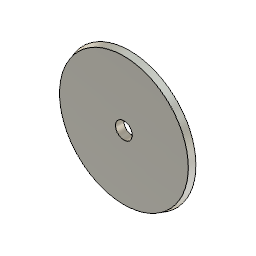
Ensamble v3 (Autodesk Fusion 360 archive; units mm, degrees)
design "Anillo de engrane 2"
Autodesk Fusion 360 part; units mm, degrees
sketch "Boceto1" plane through (0, 0, 0) normal (0, 0, 1) x (1, 0, 0)
  line L0 (0, 0) -> (17.25, 0)
  line L1 (17.25, 0) -> (17.7374, 1.5868)
  line L2 (17.7374, 1.5868) -> (15.6725, 2.221)
  line L3 (15.6725, 2.221) -> (0, 2.221)
  line L4 (0, 2.221) -> (0, 0)
  line L5 (0, 1.5868) -> (17.7374, 1.5868) construction
  dimension "d1" = 17.25
  dimension "d3" = 1.66
  dimension "d4" = 2.16
  dimension "d16" = 90
  dimension "d22" = 2.221
  constraint coincident L0.start L4.end
  constraint horizontal L0
  constraint parallel L0 L3
  constraint perpendicular L0 L4
  constraint coincident L4 L5.start
  constraint perpendicular L4 L5
  measures "d1" distance of L0.start L0.end
  measures "d3" distance of L0.end L1.end
  measures "d4" distance of L1.end L2.end
  measures "d16" angle of L1 L2
  measures "d22" distance of L0 L3
revolve "Revolución2" add sketch "Boceto1" angle 360 about axis through (0, 2.221, 0) along (0, -1, 0)
sketch "Boceto4" plane through (0, 0, 0) normal (0, -1, 0) x (1, 0, 0)
  circle A0 centre (0, 0) radius 17.25
  circle A1 centre (0, 0) radius 2.25
  dimension "d19" = 4.5
  constraint coincident A0.centre A1.centre
  measures "d19" diameter of A1
extrude "Extruir3" cut sketch "Boceto4" along normal mid plane 26 contours A1

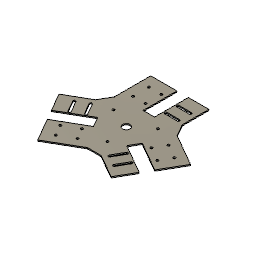
design "Robot Delta base"
Autodesk Fusion 360 part; units mm, degrees
sketch "Boceto1" plane through (0, 0, 0) normal (0, 0, 1) x (1, 0, 0)
  circle A0 centre (0, 0) radius 100
  line L0 (0, 200.0885) -> (-173.2817, -100.0442)
  line L1 (-173.2817, -100.0442) -> (173.2817, -100.0442)
  line L2 (173.2817, -100.0442) -> (0, 200.0885)
  line L3 (0, -100.0442) -> (0, 200.0885) construction
  line L4 (-173.2817, -100.0442) -> (86.6408, 50.0221) construction
  line L5 (173.2817, -100.0442) -> (-86.6408, 50.0221) construction
  line L6 (51.9615, -30) -> (59.4615, -17.0096)
  line L7 (59.4615, -17.0096) -> (128.7436, -57.0096)
  line L8 (44.4615, -42.9904) -> (113.7436, -82.9904)
  line L9 (51.9615, -30) -> (44.4615, -42.9904)
  line L10 (-15, 60) -> (-15, 140)
  line L11 (0.5917, 60) -> (15, 60)
  line L12 (15, 60) -> (15, 140)
  line L13 (-123.1844, 140) -> (49.0279, 140)
  line L14 (-15, 60) -> (0.5917, 60)
  line L15 (157.2934, 41.8591) -> (75.3655, -100.0442)
  line L16 (-44.4615, -42.9904) -> (-113.7436, -82.9904)
  line L17 (-59.4615, -17.0096) -> (-128.7436, -57.0096)
  line L18 (-30.9577, -176.4773) -> (-124.184, -15.0046)
  line L19 (-44.4615, -42.9904) -> (-59.4615, -17.0096)
  circle A1 centre (0, 0) radius 10
  line L20 (-115.5498, 0.1381) -> (-24.8334, -156.9872) construction
  line L21 (212.8999, -69.8468) -> (210.5798, -60.2903) construction
  line L22 (57.7095, -100.0442) -> (164.8904, 85.5986) construction
  line L23 (57.7861, 100) -> (-125, 100) construction
  line L24 (-85, 150) -> (-15, 150)
  line L25 (-15, 150) -> (-15, 50)
  line L26 (-15, 50) -> (-85, 50)
  line L27 (-85, 50) -> (-85, 150)
  circle A2 centre (45, 84) radius 3
  circle A3 centre (25, 84) radius 3
  circle A4 centre (25, 116) radius 3
  circle A5 centre (45, 116) radius 3
  line L28 (28.8663, 150.0905) -> (70, 150.0905)
  line L29 (70, 150.0905) -> (70, 78.8449)
  line L30 (21, 113) -> (55, 113)
  line L31 (21, 119) -> (55, 119)
  arc A6 (55, 113) -> (55, 119) centre (55, 116) ccw
  arc A7 (21, 119) -> (21, 113) centre (21, 116) ccw
  line L32 (21, 81) -> (55, 81)
  circle A8 centre (25, 84) radius 3
  circle A9 centre (45, 84) radius 3
  line L33 (21, 87) -> (55, 87)
  arc A10 (21, 87) -> (21, 81) centre (21, 84) ccw
  arc A11 (55, 81) -> (55, 87) centre (55, 84) ccw
  line L34 (-0.8013, -98.6122) -> (-87.4038, -148.6122)
  line L35 (-35.8013, -37.9904) -> (-0.8013, -98.6122)
  line L36 (-44.4615, -42.9904) -> (-113.7436, -82.9904)
  line L37 (-122.4038, -87.9904) -> (-35.8013, -37.9904)
  line L38 (-87.4038, -148.6122) -> (-122.4038, -87.9904)
  line L39 (-59.6514, -176.6808) -> (-145.7575, -27.5406)
  line L40 (-59.4615, -17.0096) -> (-128.7436, -57.0096)
  line L41 (-52.2574, -29.4875) -> (-59.4615, -17.0096)
  line L42 (-44.4615, -42.9904) -> (-52.2574, -29.4875)
  line L43 (-80.6481, -22.3135) -> (-97.6481, 7.1314)
  circle A12 centre (-112.9589, -36.3494) radius 3
  circle A13 centre (-122.9589, -19.0289) radius 3
  circle A14 centre (-85.2461, -20.3494) radius 3
  circle A15 centre (-95.2461, -3.0289) radius 3
  line L44 (-85.8442, -25.3135) -> (-102.8442, 4.1314)
  arc A16 (-85.8442, -25.3135) -> (-80.6481, -22.3135) centre (-83.2461, -23.8135) ccw
  arc A17 (-97.6481, 7.1314) -> (-102.8442, 4.1314) centre (-100.2461, 5.6314) ccw
  arc A18 (-113.557, -41.3135) -> (-108.3609, -38.3135) centre (-110.9589, -39.8135) ccw
  line L45 (-108.3609, -38.3135) -> (-125.3609, -8.8686)
  line L46 (-113.557, -41.3135) -> (-130.557, -11.8686)
  arc A19 (-125.3609, -8.8686) -> (-130.557, -11.8686) centre (-127.9589, -10.3686) ccw
  line L47 (-144.4154, -50.0463) -> (-164.9822, -14.4235)
  line L48 (-164.9822, -14.4235) -> (-103.2817, 21.1993)
  line L49 (85.8013, 48.6122) -> (172.4038, -1.3878)
  line L50 (50.8013, -12.0096) -> (85.8013, 48.6122)
  line L51 (59.4615, -17.0096) -> (128.7436, -57.0096)
  line L52 (137.4038, -62.0096) -> (50.8013, -12.0096)
  line L53 (172.4038, -1.3878) -> (137.4038, -62.0096)
  line L54 (182.8357, 36.6808) -> (96.7296, -112.4594)
  line L55 (44.4615, -42.9904) -> (113.7436, -82.9904)
  line L56 (51.6657, -30.5125) -> (44.4615, -42.9904)
  line L57 (59.4615, -17.0096) -> (51.6657, -30.5125)
  line L58 (59.6481, -58.6865) -> (42.6481, -88.1314)
  circle A20 centre (87.9589, -79.6506) radius 3
  circle A21 centre (77.9589, -96.9711) radius 3
  circle A22 centre (60.2461, -63.6506) radius 3
  circle A23 centre (50.2461, -80.9711) radius 3
  line L59 (64.8442, -61.6865) -> (47.8442, -91.1314)
  arc A24 (64.8442, -61.6865) -> (59.6481, -58.6865) centre (62.2461, -60.1865) ccw
  arc A25 (42.6481, -88.1314) -> (47.8442, -91.1314) centre (45.2461, -89.6314) ccw
  arc A26 (92.557, -77.6865) -> (87.3609, -74.6865) centre (89.9589, -76.1865) ccw
  line L60 (87.3609, -74.6865) -> (70.3609, -104.1314)
  line L61 (92.557, -77.6865) -> (75.557, -107.1314)
  arc A27 (70.3609, -104.1314) -> (75.557, -107.1314) centre (72.9589, -105.6314) ccw
  line L62 (115.549, -100.0442) -> (94.9822, -135.667)
  line L63 (94.9822, -135.667) -> (33.2817, -100.0442)
  line L64 (-15, 150) -> (28.8663, 150.0905)
  line L65 (15, 150.0619) -> (15, 140)
  line L66 (-144.4154, -50.0463) -> (-122.4038, -87.9904)
  line L67 (115.549, -100.0442) -> (137.4038, -62.0096)
  line L68 (122.3417, -88.2227) -> (113.7436, -82.9904)
  line L69 (-137.4729, -62.0138) -> (-128.7436, -57.0096)
  circle A28 centre (118.8973, -36.3138) radius 3
  circle A29 centre (135.4123, -7.709) radius 3
  circle A30 centre (98.8228, 13.416) radius 3
  circle A31 centre (82.3078, -15.1888) radius 3
  circle A32 centre (-61.03, 121.125) radius 3
  circle A33 centre (-28, 121.125) radius 3
  circle A34 centre (-28, 78.875) radius 3
  circle A35 centre (-61.03, 78.875) radius 3
  circle A36 centre (-74.3823, -113.416) radius 3
  circle A37 centre (-90.8973, -84.8112) radius 3
  circle A38 centre (-54.3078, -63.6862) radius 3
  circle A39 centre (-37.7928, -92.291) radius 3
  line L70 (-3.1207, -99.9513) -> (33.2817, -100.0442)
  line L71 (-103.2817, 21.1993) -> (-85, 52.8641)
  line L72 (0, 0) -> (15.0803, -100.0442) construction
  circle A40 centre (8.9431, -59.3298) radius 3
  circle A41 centre (0, 0) radius 60 construction
  circle A42 centre (46.9095, 37.4099) radius 3
  circle A43 centre (-55.8526, 21.9199) radius 3
  point P0 (-86.6025, -50)
  point P1 (-85.2461, -20.3494)
  point P2 (60.2461, -63.6506)
  dimension "d1" = 200
  dimension "d5" = 80
  dimension "d6" = 60
  dimension "d7" = 30
  dimension "d8" = 80
  dimension "d9" = 30
  dimension "d10" = 15
  dimension "d13" = 60
  dimension "d16" = 80
  dimension "d17" = 30
  dimension "d18" = 15
  dimension "d19" = 60
  dimension "d22" = 80
  dimension "d24" = 80
  dimension "d25" = 20
  dimension "d27" = 70
  dimension "d28" = 100
  dimension "d29" = 50
  dimension "d47" = 6
  dimension "d48" = 6
  dimension "d49" = 6
  dimension "d50" = 6
  dimension "d51" = 20
  dimension "d52" = 20
  dimension "d53" = 32
  dimension "d55" = 10
  dimension "d56" = 10
  dimension "d57" = 16
  dimension "d58" = 16
  dimension "d59" = 32
  dimension "d60" = 10
  dimension "d61" = 4
  dimension "d62" = 4
  dimension "d63" = 10
  dimension "d68" = 6
  dimension "d69" = 13
  dimension "d70" = 21.125
  dimension "d71" = 6
  dimension "d72" = 33.03
  dimension "d73" = 21.125
  dimension "d74" = 21.125
  dimension "d76" = 360
  dimension "d94" = 36.4024
  dimension "d95" = 18.201
  dimension "d96" = 6
  dimension "d98" = 60
  dimension "d99" = 120
  dimension "d101" = 360
  constraint coincident A0.centre A1.centre
  constraint midpoint L1 L3.start
  constraint perpendicular L1 L3
  constraint midpoint L2 L4.end
  constraint perpendicular L2 L4
  constraint midpoint L0 L5.end
  constraint perpendicular L0 L5
  constraint coincident L5 L6.start
  constraint perpendicular L5 L6
  constraint perpendicular L6 L7
  constraint symmetric L5 L6.start L9.start
  constraint symmetric L5 L6.end L8.start
  constraint symmetric L5 L7.end L8.end
  constraint perpendicular L12 L13
  constraint perpendicular L3 L14
  constraint perpendicular L17 L18
  constraint perpendicular L17 L19
  constraint horizontal L13
  constraint coincident L0 L18.end
  constraint coincident L1 L15.end
  constraint coincident A0 P0
  constraint coincident L4 P0
  constraint perpendicular L4 L20
  constraint tangent A0 L20
  constraint perpendicular L5 L22
  constraint tangent A0 L22
  constraint coincident L1 L22.start
  constraint equal L10 L12
  constraint coincident L2 L23.start
  constraint perpendicular L12 L23
  constraint horizontal L24
  constraint vertical L25
  constraint horizontal L26
  constraint vertical L27
  constraint coincident L2 L28.start
  constraint parallel L13 L28
  constraint coincident L2 L29.end
  constraint perpendicular L28 L29
  constraint perpendicular L3 L30
  constraint tangent A4 L31
  constraint tangent L30 A6
  constraint tangent L31 A6
  constraint tangent L30 A7
  constraint symmetric L23 A4 A8
  constraint symmetric L23 A5 A9
  constraint symmetric L23 L30.start L33.start
  constraint symmetric L23 L30.end L33.end
  constraint symmetric L23 L31.start L32.start
  constraint symmetric L23 L31.end L32.end
  constraint symmetric L23 A6 A11
  constraint symmetric L23 A7 A10
  constraint coincident L64 L65.start
  constraint perpendicular L13 L65
  constraint coincident L67 L68.start
  constraint coincident L66 L69.start
  constraint symmetric L22 A28 A31
  constraint symmetric L22 A29 A30
  constraint coincident A0 L70.start
  constraint coincident L34 L70.start
  constraint coincident L0 L71.end
  constraint coincident L27 L71.end
  constraint parallel L0 L71
  constraint coincident L1 L72.end
  constraint coincident L72 A40.centre
  constraint concentric A1 A41
  measures "d1" diameter of A0
  measures "d5" distance of L6.end L7.end
  measures "d6" distance of A0.centre L6.start
  measures "d7" distance of L7 L8
  measures "d8" distance of L10.start L10.end
  measures "d9" distance of L10 L12
  measures "d10" distance of L3 L12
  measures "d13" distance of A0.centre L14
  measures "d16" distance of L16.start L16.end
  measures "d17" distance of L16 L17
  measures "d18" distance of L4 L17
  measures "d19" distance of A0.centre L19
  measures "d22" distance of L17.start L17.end
  measures "d24" distance of L11 L13
  measures "d25" diameter of A1
  measures "d27" distance of L25 L27
  measures "d28" distance of L24.start L26.end
  measures "d29" distance of L23 L24
  measures "d47" diameter of A2
  measures "d48" diameter of A3
  measures "d49" diameter of A4
  measures "d50" diameter of A5
  measures "d51" distance of A2.centre A3.centre
  measures "d52" horizontal distance of A4.centre A5.centre
  measures "d53" vertical distance of A2.centre A5.centre
  measures "d55" distance of L12 A3.centre
  measures "d56" distance of L12 A4.centre
  measures "d57" distance of L23 A5.centre
  measures "d58" distance of L23 A4.centre
  measures "d59" distance of A3.centre A4.centre
  measures "d60" horizontal distance of A5.centre L30.end
  measures "d61" horizontal distance of A4.centre L30.start
  measures "d62" horizontal distance of A4.centre L31.start
  measures "d63" horizontal distance of A5.centre L31.end
  measures "d68" diameter of A28
  measures "d69" distance of L7 A28.centre
  measures "d70" distance of L22 A28.centre
  measures "d71" diameter of A29
  measures "d72" distance of A28.centre A29.centre
  measures "d73" distance of L22 A29.centre
  measures "d74" distance of L22 A30.centre
  measures "d94" horizontal distance of L63.end L70.start
  measures "d95" horizontal distance of L70.start L72.end
  measures "d96" diameter of A40
  measures "d98" distance of A0.centre A40.centre
  measures "d99" diameter of A41
extrude "Extruir3" add sketch "Boceto1" along normal blind 3 contours A0 L7 L49 L50 L51 L52 A30 | A0 L2 L7 L15 L49 L51 L52 A30 | A0 L1 L8 L15 L55 L59 A25 A26 L60 L70 | A0 L6 L8 L9 L11 L12 L14 L17 L19 L25 L26 L27 L32 L33 A10 A11 L34 L35 L37 L40 L41 L42 L43 L44 A16 A17 L49 L50 L52 L55 L56 L57 L58 L59 A24 A25 L70 | L2 L7 L15 L51 L52 L54 | A0 L2 L12 L13 L30 L31 A7 L33 A11 L49 | L1 L8 L15 L54 L55 A26 L61 | L2 L52 L53 L54 | L2 L15 L49 L54 | L2 L15 L49 | L1 L54 L67 L68 | L2 L49 L53 L54 | L2 L28 L29 L30 L31 A6 | L1 L60 L61 A27 L62 L63 | A0 L1 L16 L18 L34 L36 L37 A39 | A0 L16 L34 L35 L36 L37 A39 | A0 L10 L25 L26 L27 A35 | A0 L0 L10 L13 L25 L27 A35 | L2 L13 L64 L65 | L1 L18 L34 | L0 L13 L24 L25 | L1 L18 L34 L39 | L1 L16 L18 L36 L37 L39 | L0 L13 L24 L27 | L0 L13 L27 | L1 L34 L38 L39 | L1 L37 L38 L39 | A0 L0 L17 L18 L27 L40 L44 A17 A18 L45 L71 | L0 L17 L18 L39 L40 A18 L46 | L0 L45 L46 A19 L47 L48 | L0 L39 L66 L69

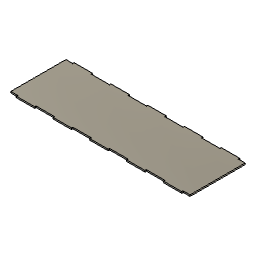
design "Parte Superior"
Autodesk Fusion 360 part; units mm, degrees
sketch "Boceto1" plane through (0, 0, 0) normal (0, 0, 1) x (1, 0, 0)
  line L0 (-195, 0) -> (-195, -60)
  line L1 (-100, -60) -> (-100, -63)
  line L2 (-100, -63) -> (-60, -63)
  line L3 (-60, -63) -> (-60, -60)
  line L4 (-60, -60) -> (-20, -60)
  line L5 (-20, -60) -> (-20, -63)
  line L6 (-20, -63) -> (0, -63)
  line L7 (0, 0) -> (-195, 0) construction
  line L8 (-100, 60) -> (-100, 63)
  line L9 (-100, 63) -> (-60, 63)
  line L10 (-20, 60) -> (-20, 63)
  line L11 (-60, 60) -> (-20, 60)
  line L12 (-60, 63) -> (-60, 60)
  line L13 (-20, 63) -> (0, 63)
  line L14 (-195, 0) -> (-195, 60)
  line L15 (0, -63) -> (0, 63) construction
  line L16 (0, -63) -> (0, 63) construction
  line L17 (-100, -60) -> (-140, -60)
  line L18 (-140, -60) -> (-140, -63)
  line L19 (-140, -63) -> (-180, -63)
  line L20 (-180, -63) -> (-180, -60)
  line L21 (-180, -60) -> (-195, -60)
  line L22 (-100, 60) -> (-140, 60)
  line L23 (-140, 60) -> (-140, 63)
  line L24 (-140, 63) -> (-180, 63)
  line L25 (-180, 63) -> (-180, 60)
  line L26 (-180, 60) -> (-195, 60)
  line L27 (60, -60) -> (20, -60)
  line L28 (100, 63) -> (60, 63)
  line L29 (60, 60) -> (20, 60)
  line L30 (0, 0) -> (195, 0) construction
  line L31 (20, 60) -> (20, 63)
  line L32 (20, 63) -> (0, 63)
  line L33 (140, -63) -> (180, -63)
  line L34 (180, -63) -> (180, -60)
  line L35 (180, -60) -> (195, -60)
  line L36 (195, 0) -> (195, -60)
  line L37 (195, 0) -> (195, 60)
  line L38 (180, 60) -> (195, 60)
  line L39 (180, 63) -> (180, 60)
  line L40 (140, 63) -> (180, 63)
  line L41 (100, -60) -> (140, -60)
  line L42 (100, -63) -> (60, -63)
  line L43 (20, -63) -> (0, -63)
  line L44 (100, 60) -> (140, 60)
  line L45 (140, 60) -> (140, 63)
  line L46 (100, -60) -> (100, -63)
  line L47 (140, -60) -> (140, -63)
  line L48 (20, -63) -> (20, -60)
  line L49 (60, -63) -> (60, -60)
  line L50 (100, 63) -> (100, 60)
  line L51 (60, 63) -> (60, 60)
  point P0 (0, 63)
  dimension "d2" = 195
  dimension "d4" = 20
  dimension "d6" = 40
  dimension "d7" = 3
  dimension "d8" = 3
  dimension "d9" = 3
  dimension "d10" = 60
  dimension "d13" = 40
  dimension "d14" = 40
  dimension "d15" = 3
  dimension "d16" = 40
  dimension "d17" = 3
  dimension "d18" = 40
  dimension "d19" = 3
  dimension "d20" = 40
  dimension "d21" = 3
  constraint vertical L0
  constraint perpendicular L1 L2
  constraint perpendicular L2 L3
  constraint perpendicular L3 L4
  constraint perpendicular L4 L5
  constraint perpendicular L5 L6
  constraint coincident L7.start L30.start
  constraint perpendicular L0 L7
  constraint symmetric L0.start L7 L14.start
  constraint symmetric L0.end L7 L14.end
  constraint symmetric L1.start L7 L8.start
  constraint symmetric L1.end L7 L8.end
  constraint symmetric L2.end L7 L9.end
  constraint symmetric L3.end L7 L11.start
  constraint symmetric L4.end L7 L10.start
  constraint symmetric L5.end L7 L10.end
  constraint symmetric P0 L15 L13.end
  constraint perpendicular L1 L17
  constraint perpendicular L17 L18
  constraint perpendicular L18 L19
  constraint perpendicular L19 L20
  constraint perpendicular L0 L21
  constraint perpendicular L8 L22
  constraint perpendicular L22 L23
  constraint perpendicular L23 L24
  constraint perpendicular L24 L25
  constraint symmetric L0.start L15 L30.end
  constraint symmetric L0.end L15 L35.end
  constraint symmetric L1.start L15 L41.start
  constraint symmetric L1.end L15 L42.start
  constraint symmetric L2.end L15 L42.end
  constraint symmetric L3.end L15 L27.start
  constraint symmetric L4.end L15 L27.end
  constraint symmetric L5.end L15 L43.start
  constraint symmetric L6.end L15 L16.start
  constraint symmetric L7.start L15 L30.start
  constraint symmetric L8.start L15 L44.start
  constraint symmetric L11.start L15 L29.start
  constraint symmetric L9.end L15 L28.end
  constraint symmetric L8.end L15 L28.start
  constraint symmetric L10.start L15 L29.end
  constraint symmetric L14.end L15 L37.end
  constraint symmetric L10.end L15 L31.end
  constraint symmetric L15 P0 L13.end
  constraint symmetric L15 L17.end L41.end
  constraint symmetric L15 L18.end L33.start
  constraint symmetric L15 L19.end L33.end
  constraint symmetric L15 L20.end L34.end
  constraint symmetric L15 L22.end L44.end
  constraint symmetric L15 L23.end L40.start
  constraint symmetric L15 L24.end L39.start
  constraint symmetric L15 L25.end L38.start
  measures "d2" distance of L0.start L7.start
  measures "d4" distance of L5.end L6.end
  measures "d6" distance of L1.end L2.end
  measures "d7" distance of L1.start L1.end
  measures "d8" distance of L2.end L3.end
  measures "d9" distance of L4.end L5.end
  measures "d10" distance of L0.start L0.end
  measures "d13" distance of L3.end L4.end
  measures "d14" distance of L1.start L17.end
  measures "d15" distance of L17.end L18.end
  measures "d16" distance of L18.end L19.end
  measures "d17" distance of L19.end L20.end
  measures "d18" distance of L8.start L22.end
  measures "d19" distance of L22.end L23.end
  measures "d20" distance of L23.end L24.end
  measures "d21" distance of L24.end L25.end
extrude "Extruir2" add sketch "Boceto1" along normal blind 3

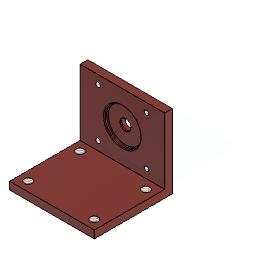
design "SoporteNEMA17 v10"
Autodesk Fusion 360 part; units mm, degrees
sketch "Sketch1" plane through (0, 0, 0) normal (0, 0, 1) x (1, 0, 0)
  line L0 (21.125, 21.125) -> (-21.125, 21.125)
  line L1 (-21.125, 21.125) -> (-21.125, -21.125)
  line L2 (-21.125, -21.125) -> (21.125, -21.125)
  line L3 (21.125, -21.125) -> (21.125, 21.125)
  line L4 (21.125, 21.125) -> (-21.125, -21.125) construction
  line L5 (-21.125, 21.125) -> (21.125, -21.125) construction
  dimension "d1" = 42.25
  dimension "d2" = 42.25
  constraint horizontal L0
  constraint perpendicular L0 L1
  constraint parallel L0 L2
  constraint parallel L1 L3
  constraint coincident L4 origin
  constraint coincident L5 origin
  measures "d1" distance of L1.end L2.end
  measures "d2" distance of L0.end L1.end
extrude "Extrude1" add sketch "Sketch1" along normal blind 5
sketch "Sketch2" plane through (0, 0, 5) normal (0, 0, 1) x (-1, 0, 0)
  line L0 (-21.125, 21.125) -> (-21.125, -21.125)
  line L1 (-21.125, -21.125) -> (21.125, -21.125)
  line L2 (21.125, -21.125) -> (21.125, 21.125)
  line L3 (21.125, 21.125) -> (-21.125, 21.125)
  circle A0 centre (0, 0) radius 11.5
  line L4 (-21.125, 0) -> (21.125, 0) construction
  line L5 (0, -21.125) -> (0, 21.125) construction
  point P0 (-15.5, -15.5)
  point P1 (15.5, -15.5)
  point P2 (-15.5, 15.5)
  point P3 (15.5, 15.5)
  dimension "d5" = 23
  dimension "d32" = 5.625
  dimension "d33" = 5.625
  constraint coincident A0.centre origin
  constraint midpoint L0 L4.start
  constraint midpoint L2 L4.end
  constraint midpoint L1 L5.start
  constraint midpoint L3 L5.end
  constraint symmetric P0 L5 P1
  constraint symmetric P0 L4 P2
  constraint symmetric L4 P1 P3
  measures "d5" diameter of A0
  measures "d32" distance of L0 P0
  measures "d33" distance of L1 P0
extrude "Extrude2" cut sketch "Sketch2" against normal blind 2 contours A0
sketch "Sketch3" plane through (0, 0, 3) normal (0, 0, 1) x (-1, 0, 0)
  circle A0 centre (0, 0) radius 11.5
  circle A1 centre (0, 0) radius 3
  dimension "d8" = 6
  constraint coincident A0.centre A1.centre
  measures "d8" diameter of A1
extrude "Extrude3" cut sketch "Sketch3" against normal blind 3 contours A1
sketch "Sketch6" plane through (0, 0, 0) normal (0, 0, -1) x (1, 0, 0)
  circle A0 centre (0, 0) radius 3
  line L0 (21.125, -21.125) -> (21.125, 21.125)
  line L1 (21.125, 21.125) -> (-21.125, 21.125)
  line L2 (-21.125, 21.125) -> (-21.125, -21.125)
  line L3 (-21.125, -21.125) -> (21.125, -21.125)
extrude "Extrude4" add 1 faces at (-7.0417, -21.125, 1.6667) along direction (0, -1, 0) blind 5
sketch "Sketch5" plane through (0, 0, 5) normal (0, 0, 1) x (-1, 0, 0)
  circle A0 centre (0, 0) radius 11.5
  line L0 (-21.125, 26.125) -> (-21.125, -21.125)
  line L1 (-21.125, -21.125) -> (21.125, -21.125)
  line L2 (21.125, -21.125) -> (21.125, 26.125)
  line L3 (21.125, 26.125) -> (-21.125, 26.125)
  line L4 (21.125, 23.625) -> (-21.125, 23.625)
  line L5 (21.125, -21.125) -> (-21.125, -21.125)
  line L6 (-21.125, -21.125) -> (-21.125, 21.125)
  dimension "d15" = 2.5
  constraint coincident L2 L4.start
  constraint coincident L0 L4.end
  constraint perpendicular L0 L4
  measures "d15" distance of L3 L4
extrude "Extrude5" add sketch "Sketch5" along normal blind 34 contours L0 L2 L3 L4
fillet "Fillet1" radius 0.5 2 faces at (-8.6127, 0.7204, 3) (-11.4857, 0.5732, 3.6667)
sketch "Sketch11" plane through (0, 0, 0) normal (0, 0, -1) x (1, 0, 0)
  line L0 (0, -0.125) -> (0, -42.125) construction
  line L1 (21.1283, 0) -> (-21.125, 0) construction
  line L2 (21.125, -21.125) -> (21.125, 21.125)
  line L3 (-21.125, -21.125) -> (21.125, -21.125)
  line L4 (-21.125, 21.125) -> (-21.125, -21.125)
  constraint vertical L0
  constraint perpendicular L0 L1
  constraint midpoint L0 L3
  constraint midpoint L1.end L4
hole "Hole2" at (15.5, 15.5, 0) at (-15.5, 15.5, 0) at (-15.5, -15.5, 0) at (15.5, -15.5, 0) direction (0, 0, 1) diameter 3.4 depth 5 tip angle 118 counterbore diameter 6.5 counterbore depth 3
move_body "Move1" bodies 1 to x (1, 0, 0) y (0, 0, 1) z (0, -1, 0) at (0, -26.125, 26.125)
extrude "Extrude6" cut 1 faces at (7.0417, -65.125, 1.6667) along direction (0, 1, 0) blind 6.139
extrude "Extrude7" add 1 faces at (-7.0417, -40.412, 2.5) along direction (0, 0, 1) blind 2.5
sketch "Sketch14" plane through (0, 0, 5) normal (0, 0, 1) x (-1, 0, 0)
  line L0 (21.125, 58.986) -> (-21.125, 58.986)
  line L1 (-21.125, 58.986) -> (-21.125, 31.125)
  line L2 (-21.125, 31.125) -> (21.125, 31.125)
  line L3 (21.125, 31.125) -> (21.125, 58.986)
  line L4 (-21.125, 45.0555) -> (21.125, 45.0555) construction
  line L5 (0, 58.986) -> (0, 31.125) construction
  circle A0 centre (17.125, 35.125) radius 1.5
  circle A1 centre (17.125, 54.986) radius 1.5
  circle A2 centre (-17.125, 35.125) radius 1.5
  circle A3 centre (-17.125, 54.986) radius 1.5
  dimension "d82" = 3
  dimension "d83" = 4
  dimension "d84" = 4
  dimension "d85" = 3
  dimension "d86" = 4
  dimension "d87" = 4
  dimension "d88" = 3
  dimension "d89" = 3
  dimension "d90" = 4
  dimension "d91" = 4
  dimension "d92" = 4
  dimension "d93" = 4
  constraint midpoint L1 L4.start
  constraint midpoint L3 L4.end
  constraint midpoint L0 L5.start
  constraint midpoint L2 L5.end
  measures "d82" diameter of A0
  measures "d83" distance of L2 A0.centre
  measures "d84" distance of L3 A0.centre
  measures "d85" diameter of A1
  measures "d86" distance of L3 A1.centre
  measures "d87" distance of L0 A1.centre
  measures "d88" diameter of A2
  measures "d89" diameter of A3
  measures "d90" distance of L1 A2.centre
  measures "d91" distance of L2 A2.centre
  measures "d92" distance of L1 A3.centre
  measures "d93" distance of L0 A3.centre
extrude "Extruir14" add 1 faces at (-21.125, -27.7917, 17.4167) along direction (-1, 0, 0) blind 6
extrude "Extruir15" add 1 faces at (21.125, -27.7917, 17.4167) along direction (1, 0, 0) blind 6
extrude "Extruir16" add 1 faces at (-9.0417, -58.986, 3.3333) along direction (0, -1, 0) blind 17.169
sketch "Boceto17" plane through (0, 0, 5) normal (0, 0, 1) x (-1, 0, 0)
  line L0 (-27.125, 76.155) -> (-27.125, 31.125)
  line L1 (-27.125, 31.125) -> (27.125, 31.125)
  line L2 (27.125, 31.125) -> (27.125, 76.155)
  line L3 (27.125, 76.155) -> (-27.125, 76.155)
  circle A0 centre (21.125, 37.125) radius 3
  circle A1 centre (-21.125, 37.125) radius 3
  circle A2 centre (21.125, 70.155) radius 3
  circle A3 centre (-21.125, 70.155) radius 3
  point P0 (22.3785, 34.6118)
  dimension "d100" = 6
  dimension "d101" = 6
  dimension "d102" = 6
  dimension "d103" = 6
  dimension "d104" = 6
  dimension "d105" = 6
  dimension "d106" = 6
  dimension "d107" = 6
  dimension "d108" = 6
  dimension "d109" = 6
  dimension "d110" = 6
  dimension "d111" = 6
  measures "d100" diameter of A0
  measures "d101" distance of L2 A0.centre
  measures "d102" distance of L1 A0.centre
  measures "d103" diameter of A1
  measures "d104" distance of L1 A1.centre
  measures "d105" distance of L0 A1.centre
  measures "d106" diameter of A2
  measures "d107" diameter of A3
  measures "d108" distance of L2 A2.centre
  measures "d109" distance of L3 A2.centre
  measures "d110" distance of L0 A3.centre
  measures "d111" distance of L3 A3.centre
thread "Rosca5" "ISO Metric profile 3.5 M3.5x0.6 M3.5x0.6 6H" major diameter 3.5995 minor diameter 2.93 pitch 0.6 angle 60 resizes the face on face at (-15.3307, -30.4583, 43.3166)
thread "Rosca6" "ISO Metric profile 3.5 M3.5x0.6 M3.5x0.6 6H" major diameter 3.5995 minor diameter 2.93 pitch 0.6 angle 60 resizes the face on face at (15.5847, -29.7917, 43.3229)
thread "Rosca7" "ISO Metric profile 3.5 M3.5x0.6 M3.5x0.6 6H" major diameter 3.5995 minor diameter 2.93 pitch 0.6 angle 60 resizes the face on face at (-15.4153, -29.7917, 12.3229)
thread "Rosca8" "ISO Metric profile 3.5 M3.5x0.6 M3.5x0.6 6H" major diameter 3.5995 minor diameter 2.93 pitch 0.6 angle 60 resizes the face on face at (15.5847, -29.7917, 12.3229)
extrude "Extruir18" cut sketch "Boceto17" against normal blind 29 contours A0 | A1 | A2 | A3
thread "Rosca9" "ISO Metric profile 6.0 M6x1 M6x1 6H" major diameter 6.147 minor diameter 5.035 pitch 1 angle 60 resizes the face on face at (-18.1399, -36.8263, 1.6667)
thread "Rosca10" "ISO Metric profile 6.0 M6x1 M6x1 6H" major diameter 6.147 minor diameter 5.035 pitch 1 angle 60 resizes the face on face at (24.1101, -36.8263, 1.6667)
thread "Rosca11" "ISO Metric profile 6.0 M6x1 M6x1 6H" major diameter 6.147 minor diameter 5.035 pitch 1 angle 60 resizes the face on face at (-23.6849, -71.7193, 1.6667)
thread "Rosca12" "ISO Metric profile 6.0 M6x1 M6x1 6H" major diameter 6.147 minor diameter 5.035 pitch 1 angle 60 resizes the face on face at (18.5651, -71.7193, 1.6667)

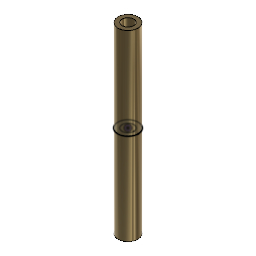
design "Union de brazo a motor"
Autodesk Fusion 360 part; units mm, degrees
sketch "Boceto1" plane through (0, 0, 0) normal (0, 0, 1) x (1, 0, 0)
  circle A0 centre (0, 0) radius 5.5
  circle A1 centre (0, 0) radius 3.175
  dimension "d1" = 11
  dimension "d2" = 6.35
  constraint coincident A0.centre A1.centre
  constraint concentric A0 A1
  measures "d1" diameter of A0
  measures "d2" diameter of A1
extrude "Extruir1" add sketch "Boceto1" along normal mid plane 100 makes body 1
extrude "Extruir2" add sketch "Boceto1" against normal blind 50 separate body contours A1 makes body 2
extrude "Extruir3" add sketch "Boceto1" along normal blind 30.95 contours A1 bodies 1 2

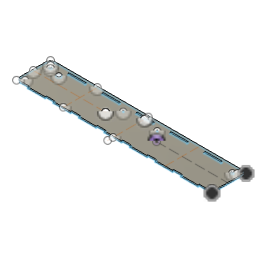
design "Lateral son motor"
Autodesk Fusion 360 part; units mm, degrees
sketch "Boceto1" plane through (0, 0, 0) normal (0, 0, 1) x (1, 0, 0)
  line L0 (-60.0005, 40.4137) -> (-60.0005, -55) construction
  line L1 (169.9995, -29.5863) -> (169.9995, 30.4137)
  line L2 (159.9995, 40.4137) -> (-60.0005, 40.4137)
  line L3 (0, 0) -> (169.9995, 0) construction
  line L4 (-0.0005, 34.4137) -> (39.9995, 34.4137)
  line L5 (39.9995, 34.4137) -> (39.9995, 31.4137)
  line L6 (39.9995, 31.4137) -> (-0.0005, 31.4137)
  line L7 (-0.0005, 31.4137) -> (-0.0005, 34.4137)
  line L8 (-60.0005, 34.4137) -> (-40.0005, 34.4137)
  line L9 (-40.0005, 34.4137) -> (-40.0005, 31.4137)
  line L10 (-40.0005, 31.4137) -> (-60.0005, 31.4137)
  circle A0 centre (-20.0005, 21.4137) radius 1
  circle A1 centre (153.9995, 24.4137) radius 2.5
  arc A2 (169.9995, 30.4137) -> (159.9995, 40.4137) centre (159.9995, 30.4137) ccw
  line L11 (79.9995, -39.5863) -> (79.9995, -42.5863)
  line L12 (79.9995, -42.5863) -> (39.9995, -42.5863)
  line L13 (39.9995, -42.5863) -> (39.9995, -39.5863)
  line L14 (39.9995, -39.5863) -> (19.9995, -39.5863)
  line L15 (19.9995, -39.5863) -> (19.9995, -42.5863)
  line L16 (19.9995, -42.5863) -> (-20.0005, -42.5863)
  line L17 (-20.0005, -42.5863) -> (-20.0005, -39.5863)
  line L18 (-20.0005, -39.5863) -> (-40.0005, -39.5863)
  line L19 (-40.0005, -39.5863) -> (-40.0005, -42.5863)
  line L20 (-40.0005, -42.5863) -> (-60.0005, -42.5863)
  line L21 (79.9995, -39.5863) -> (99.9995, -39.5863)
  line L22 (99.9995, -39.5863) -> (99.9995, -42.5863)
  line L23 (99.9995, -42.5863) -> (139.9995, -42.5863)
  line L24 (139.9995, -42.5863) -> (139.9995, -39.5863)
  line L25 (139.9995, -39.5863) -> (159.9995, -39.5863)
  arc A3 (159.9995, -39.5863) -> (169.9995, -29.5863) centre (159.9995, -29.5863) ccw
  line L26 (59.9995, 40.4137) -> (59.9995, -39.5863) construction
  line L27 (79.9995, 31.4137) -> (119.9995, 31.4137)
  line L28 (119.9995, 31.4137) -> (119.9995, 34.4137)
  line L29 (79.9995, 34.4137) -> (79.9995, 31.4137)
  line L30 (119.9995, 34.4137) -> (79.9995, 34.4137)
  line L31 (-80.0005, -39.5863) -> (-80.0005, -42.5863)
  line L32 (-120.0005, 34.4137) -> (-160.0005, 34.4137)
  line L33 (-120.0011, 0) -> (-290.0005, 0) construction
  line L34 (-60.0005, 34.4137) -> (-80.0005, 34.4137)
  line L35 (-80.0005, -42.5863) -> (-60.0005, -42.5863)
  line L36 (-290.0005, -29.5863) -> (-290.0005, 30.4137)
  line L37 (-240.0005, 34.4137) -> (-200.0005, 34.4137)
  line L38 (-200.0005, 31.4137) -> (-240.0005, 31.4137)
  line L39 (-140.0005, -42.5863) -> (-100.0005, -42.5863)
  line L40 (-160.0005, 31.4137) -> (-120.0005, 31.4137)
  line L41 (-180.0005, 40.4137) -> (-180.0005, -39.5863) construction
  line L42 (-120.0005, 31.4137) -> (-120.0005, 34.4137)
  line L43 (-80.0005, 34.4137) -> (-80.0005, 31.4137)
  line L44 (-200.0005, 34.4137) -> (-200.0005, 31.4137)
  line L45 (-160.0005, 34.4137) -> (-160.0005, 31.4137)
  arc A4 (-280.0005, 40.4137) -> (-290.0005, 30.4137) centre (-280.0005, 30.4137) ccw
  circle A5 centre (-274.0005, 24.4137) radius 2.5
  line L46 (-240.0005, 31.4137) -> (-240.0005, 34.4137)
  line L47 (-140.0005, -39.5863) -> (-140.0005, -42.5863)
  line L48 (-160.0005, -39.5863) -> (-140.0005, -39.5863)
  line L49 (-160.0005, -42.5863) -> (-160.0005, -39.5863)
  line L50 (-100.0005, -42.5863) -> (-100.0005, -39.5863)
  line L51 (-200.0005, -42.5863) -> (-160.0005, -42.5863)
  line L52 (-220.0005, -39.5863) -> (-220.0005, -42.5863)
  line L53 (-200.0005, -39.5863) -> (-220.0005, -39.5863)
  line L54 (-280.0005, 40.4137) -> (-60.0005, 40.4137)
  line L55 (-200.0005, -39.5863) -> (-200.0005, -42.5863)
  line L56 (-100.0005, -39.5863) -> (-80.0005, -39.5863)
  line L57 (-260.0005, -39.5863) -> (-280.0005, -39.5863)
  line L58 (-260.0005, -42.5863) -> (-260.0005, -39.5863)
  arc A6 (-290.0005, -29.5863) -> (-280.0005, -39.5863) centre (-280.0005, -29.5863) ccw
  line L59 (-220.0005, -42.5863) -> (-260.0005, -42.5863)
  line L60 (-80.0005, 31.4137) -> (-60.0005, 31.4137)
  circle A7 centre (-100.0005, 21.4137) radius 1
  circle A8 centre (-247.8005, 17.7137) radius 5
  point P0 (169.9995, -39.5863)
  point P1 (169.9995, 40.4137)
  point P2 (-120.0011, 0)
  point P3 (-290.0005, 40.4137)
  point P4 (-290.0005, -39.5863)
  point P5 (-120.0011, 0)
  dimension "d4" = 80
  dimension "d16" = 40
  dimension "d18" = 6
  dimension "d26" = 3
  dimension "d30" = 6
  dimension "d36" = 2
  dimension "d37" = 19
  dimension "d39" = 5
  dimension "d41" = 16
  dimension "d46" = 10
  dimension "d57" = 3
  dimension "d58" = 40
  dimension "d59" = 3
  dimension "d60" = 20
  dimension "d61" = 3
  dimension "d62" = 40
  dimension "d63" = 3
  dimension "d64" = 20
  dimension "d65" = 3
  dimension "d66" = 230
  dimension "d69" = 20
  dimension "d70" = 20
  dimension "d71" = 3
  dimension "d72" = 40
  dimension "d73" = 3
  dimension "d74" = 10
  dimension "d75" = 20
  dimension "d76" = 3
  dimension "d77" = 20
  dimension "d78" = 20
  dimension "d79" = 40
  dimension "d80" = 20
  dimension "d81" = 16
  dimension "d82" = 10
  dimension "d83" = 42.2
  dimension "d84" = 22.7
  constraint vertical L0
  constraint perpendicular L0 L2
  constraint coincident L3.start origin
  constraint horizontal L3
  constraint horizontal L4
  constraint vertical L5
  constraint horizontal L6
  constraint vertical L7
  constraint horizontal L8
  constraint vertical L9
  constraint horizontal L10
  constraint coincident L0 L8.start
  constraint symmetric L3.start L0 P5
  constraint coincident L1 L3.end
  constraint coincident P1 L2
  constraint coincident P1 L1
  constraint tangent L2 A2
  constraint tangent L1 A2
  constraint coincident P0 L1
  constraint perpendicular L11 L12
  constraint perpendicular L12 L13
  constraint perpendicular L13 L14
  constraint perpendicular L14 L15
  constraint perpendicular L15 L16
  constraint perpendicular L16 L17
  constraint perpendicular L17 L18
  constraint perpendicular L18 L19
  constraint coincident L0 L20.end
  constraint perpendicular L0 L20
  constraint perpendicular L11 L21
  constraint perpendicular L21 L22
  constraint perpendicular L22 L23
  constraint perpendicular L23 L24
  constraint perpendicular L24 L25
  constraint tangent L25 A3
  constraint tangent L1 A3
  constraint coincident L2 L26.start
  constraint coincident L21 L26.end
  constraint perpendicular L21 L26
  constraint symmetric L4.start L26 L28.end
  constraint symmetric L4.end L26 L29.start
  constraint symmetric L5.end L26 L27.start
  constraint symmetric L6.end L26 L27.end
  constraint symmetric L2.end L0 L54.end
  constraint symmetric L0 P0 P4
  constraint symmetric L0 P1 P3
  constraint symmetric L0 L3.start P2
  constraint symmetric L0 L3.end L33.end
  constraint symmetric L0 L11.start L53.start
  constraint symmetric L0 L4.start L32.start
  constraint symmetric L0 L4.end L32.end
  constraint symmetric L0 L5.end L40.start
  constraint symmetric L0 L6.end L40.end
  constraint symmetric L0 L8.start L34.start
  constraint symmetric L0 L8.end L34.end
  constraint symmetric L0 L9.end L43.end
  constraint symmetric L0 L10.end L60.end
  constraint symmetric L0 A0 A7
  constraint symmetric L0 A1 A5
  constraint symmetric L0 L2.start A4.start
  constraint symmetric L0 L1.end L36.end
  constraint symmetric L0 A2 A4
  constraint symmetric L0 L11.end L51.start
  constraint symmetric L0 L12.end L49.start
  constraint symmetric L0 L13.end L48.start
  constraint symmetric L0 L14.end L47.start
  constraint symmetric L0 L15.end L39.start
  constraint symmetric L0 L16.end L39.end
  constraint symmetric L0 L17.end L50.end
  constraint symmetric L0 L18.end L31.start
  constraint symmetric L0 L19.end L31.end
  constraint symmetric L0 L20.end L35.end
  constraint symmetric L0 L21.end L52.start
  constraint symmetric L0 L22.end L52.end
  constraint symmetric L0 L23.end L58.start
  constraint symmetric L0 L24.end L57.start
  constraint symmetric L0 L25.end L57.end
  constraint symmetric L0 L1.start L36.start
  constraint symmetric L0 A3 A6
  constraint symmetric L0 L26.start L41.start
  constraint symmetric L0 L26.end L41.end
  constraint symmetric L0 L29.start L37.end
  constraint symmetric L0 L27.end L38.end
  constraint symmetric L0 L27.start L38.start
  constraint symmetric L0 L28.end L37.start
  measures "d4" distance of P0 P1
  measures "d16" distance of L4.start L4.end
  measures "d18" distance of L2 L4
  measures "d26" distance of L4.end L5.end
  measures "d30" distance of L2 L8
  measures "d36" diameter of A0
  measures "d37" distance of L2 A0.centre
  measures "d39" diameter of A1
  measures "d41" distance of L2 A1.centre
  measures "d46" radius of A2
  measures "d57" distance of L11.start L11.end
  measures "d58" distance of L11.end L12.end
  measures "d59" distance of L12.end L13.end
  measures "d60" distance of L13.end L14.end
  measures "d61" distance of L14.end L15.end
  measures "d62" distance of L15.end L16.end
  measures "d63" distance of L16.end L17.end
  measures "d64" distance of L17.end L18.end
  measures "d65" distance of L18.end L19.end
  measures "d66" distance of L0 L1
  measures "d69" distance of L19.end L20.end
  measures "d70" distance of L11.start L21.end
  measures "d71" distance of L21.end L22.end
  measures "d72" distance of L22.end L23.end
  measures "d73" distance of L23.end L24.end
  measures "d74" radius of A3
  measures "d75" distance of L8.start L8.end
  measures "d76" distance of L8.end L9.end
  measures "d77" distance of L9.end L10.end
  measures "d78" distance of L9 A0.centre
  measures "d79" distance of L7 L9
  measures "d80" distance of L5 L26
  measures "d81" distance of L1 A1.centre
  measures "d82" diameter of A8
  measures "d83" distance of L36 A8.centre
  measures "d84" distance of L54 A8.centre
extrude "Extruir7" add sketch "Boceto1" along normal blind 3

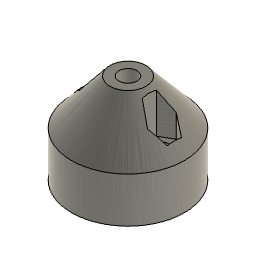
design "Como de conexion"
Autodesk Fusion 360 part; units mm, degrees
sketch "Boceto1" plane through (0, 0, 0) normal (0, 0, 1) x (1, 0, 0)
  circle A0 centre (0, 0) radius 12.5
  line L0 (12.5, 0) -> (-12.5, 0) construction
  circle A1 centre (0, 0) radius 4 construction
  circle A2 centre (0, 0) radius 2 construction
  circle A3 centre (7.5, 0) radius 1.5
  circle A4 centre (-7.5, 0) radius 1.5
  line L1 (7.5, -3.1754) -> (10.25, -1.5877)
  line L2 (10.25, -1.5877) -> (10.25, 1.5877)
  line L3 (10.25, 1.5877) -> (7.5, 3.1754)
  line L4 (7.5, 3.1754) -> (4.75, 1.5877)
  line L5 (4.75, 1.5877) -> (4.75, -1.5877)
  line L6 (4.75, -1.5877) -> (7.5, -3.1754)
  line L7 (-7.5, -3.1754) -> (-4.75, -1.5877)
  line L8 (-4.75, -1.5877) -> (-4.75, 1.5877)
  line L9 (-4.75, 1.5877) -> (-7.5, 3.1754)
  line L10 (-7.5, 3.1754) -> (-10.25, 1.5877)
  line L11 (-10.25, 1.5877) -> (-10.25, -1.5877)
  line L12 (-10.25, -1.5877) -> (-7.5, -3.1754)
  point P0 (7.5, 0)
  point P1 (-7.5, 0)
  dimension "d1" = 25
  dimension "d9" = 8
  dimension "d10" = 4
  dimension "d11" = 3
  dimension "d12" = 3
  dimension "d13" = 2.75
  dimension "d14" = 2.75
  dimension "d29" = 7.5
  dimension "d30" = 7.5
  constraint coincident A0.centre A1.centre
  constraint coincident A0 L0.start
  constraint coincident A0 L0.end
  constraint horizontal L0
  constraint concentric A1 A2
  constraint coincident L0 P0
  constraint coincident L0 P1
  constraint coincident P0 A3.centre
  constraint coincident P1 A4.centre
  constraint perpendicular L0 L11
  constraint perpendicular L0 L5
  measures "d1" diameter of A0
  measures "d9" diameter of A1
  measures "d10" diameter of A2
  measures "d11" diameter of A3
  measures "d12" diameter of A4
  measures "d13" distance of P0 L6
  measures "d14" distance of P1 L12
  measures "d29" distance of A0.centre P1
  measures "d30" distance of A0.centre P0
extrude "Extruir1" add sketch "Boceto1" against normal blind 10 contours A0 | A3 | A4 | L1 L2 L3 L4 L5 L6 | L7 L8 L9 L10 L11 L12
ref_plane "PlanoDeObra1" through (0, 0, 10) normal (0, 0, 1) x (1, 0, 0)
sketch "Boceto2" plane through (0, 0, 10) normal (0, 0, 1) x (1, 0, 0)
  circle A0 centre (0, 0) radius 12.5
  circle A1 centre (0, 0) radius 4
  dimension "d5" = -8.5
loft "Solevación1" add profiles "Boceto2" section 1 contours A1 section 2 face at (-3.3879, -0.621, 0)
sketch "Boceto3" plane through (0, 0, 10) normal (0, 0, 1) x (-1, 0, 0)
  circle A0 centre (0, 0) radius 4
  circle A1 centre (0, 0) radius 2
  dimension "d6" = 4
  constraint coincident A0.centre A1.centre
  measures "d6" diameter of A1
extrude "Extruir2" cut sketch "Boceto3" along normal mid plane 78 contours A1
sketch "Boceto4" plane through (0, 0, 10) normal (0, 0, 1) x (-1, 0, 0)
  circle A0 centre (0, 0) radius 2
  circle A1 centre (0, 0) radius 4
extrude "Extruir5" cut sketch "Boceto1" along normal blind 14 contours L1 L2 L3 L4 L5 L6
extrude "Extruir6" cut sketch "Boceto1" along normal blind 29 contours A3
extrude "Extruir7" cut sketch "Boceto1" along normal mid plane 60 contours A3
extrude "Extruir8" cut sketch "Boceto1" along normal blind 25 contours L7 L8 L9 L10 L11 L12
extrude "Extruir9" cut sketch "Boceto1" along normal mid plane 52 contours A4

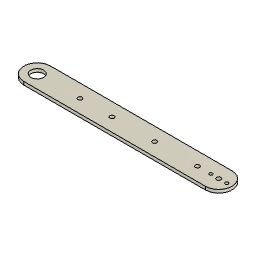
design "Brazo corto"
Autodesk Fusion 360 part; units mm, degrees
sketch "Boceto1" plane through (0, 0, 0) normal (0, 0, 1) x (1, 0, 0)
  line L0 (-85, 0) -> (85, 0)
  line L1 (-85, 25) -> (85, 25)
  line L2 (-85, 0) -> (-85, 25) construction
  line L3 (-85, 12.5) -> (85, 12.5) construction
  circle A0 centre (85, 12.5) radius 2
  arc A1 (85, 0) -> (85, 25) centre (85, 12.5) ccw
  arc A2 (-85, 25) -> (-85, 0) centre (-85, 12.5) ccw
  circle A3 centre (-85, 12.5) radius 6
  circle A4 centre (-45, 12.5) radius 2
  circle A5 centre (-15, 12.5) radius 2
  circle A6 centre (25, 12.5) radius 2
  circle A7 centre (65, 12.5) radius 2
  line L4 (85, 12.5) -> (97.5, 12.5) construction
  circle A8 centre (92.5, 12.5) radius 1.5
  circle A9 centre (77.5, 12.5) radius 1.5
  point P0 (-85, 12.5)
  dimension "d1" = 170
  dimension "d2" = 170
  dimension "d3" = 25
  dimension "d5" = 12.5
  dimension "d6" = 4
  dimension "d8" = 12
  dimension "d9" = 4
  dimension "d10" = 40
  dimension "d11" = 4
  dimension "d12" = 4
  dimension "d13" = 30
  dimension "d14" = 40
  dimension "d15" = 4
  dimension "d16" = 40
  dimension "d17" = 3
  dimension "d18" = 7.5
  dimension "d19" = 3
  dimension "d20" = 7.5
  constraint horizontal L0
  constraint midpoint origin L0
  constraint horizontal L1
  constraint coincident L2 P0
  constraint vertical L2
  constraint coincident P0 L3.start
  constraint perpendicular L2 L3
  constraint coincident L3.end A0.centre
  constraint coincident L3 A4.centre
  constraint coincident L3 A5.centre
  constraint coincident L3 A6.centre
  constraint coincident L3 A7.centre
  constraint midpoint A1 L4.end
  constraint coincident L4 A8.centre
  constraint coincident L3 A9.centre
  measures "d1" distance of L0.start L0.end
  measures "d2" distance of L1.start L1.end
  measures "d3" distance of L0 L1
  measures "d5" distance of L0.start P0
  measures "d6" diameter of A0
  measures "d8" diameter of A3
  measures "d9" diameter of A4
  measures "d10" distance of P0 A4.centre
  measures "d11" diameter of A5
  measures "d12" diameter of A6
  measures "d13" distance of A4.centre A5.centre
  measures "d14" distance of A5.centre A6.centre
  measures "d16" distance of A6.centre A7.centre
  measures "d17" diameter of A8
  measures "d18" distance of L3.end A8.centre
  measures "d19" diameter of A9
  measures "d20" distance of L3.end A9.centre
extrude "Extruir1" add sketch "Boceto1" along normal blind 3

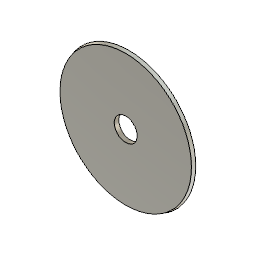
design "Anillo de engrane"
Autodesk Fusion 360 part; units mm, degrees
sketch "Boceto1" plane through (0, 0, 0) normal (0, 0, 1) x (1, 0, 0)
  line L0 (0, 0) -> (31.58, 0)
  line L1 (31.58, 0) -> (32.065, 1.5876)
  line L2 (32.065, 1.5876) -> (30, 2.2211)
  line L3 (30, 2.2211) -> (0, 2.2211)
  line L4 (0, 2.2211) -> (0, 0)
  line L5 (0, 1.5876) -> (32.065, 1.5876) construction
  dimension "d1" = 31.58
  dimension "d3" = 1.66
  dimension "d4" = 2.16
  dimension "d5" = 30
  dimension "d16" = 2.2211
  constraint coincident L0.start L4.end
  constraint horizontal L0
  constraint parallel L0 L3
  constraint perpendicular L0 L4
  constraint coincident L4 L5.start
  constraint perpendicular L4 L5
  measures "d1" distance of L0.start L0.end
  measures "d3" distance of L0.end L1.end
  measures "d4" distance of L1.end L2.end
  measures "d5" distance of L2.end L3.end
  measures "d16" distance of L0 L3
revolve "Revolución2" add sketch "Boceto1" angle 360 about axis through (0, 2.2211, 0) along (0, -1, 0)
sketch "Boceto4" plane through (0, 0, 0) normal (0, -1, 0) x (1, 0, 0)
  circle A0 centre (0, 0) radius 31.58
  circle A1 centre (0, 0) radius 5.5
  dimension "d18" = 11
  constraint coincident A0.centre A1.centre
  measures "d18" diameter of A1
extrude "Extruir3" cut sketch "Boceto4" against normal blind 39 contours A1

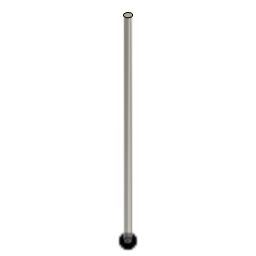
design "Barilla"
Autodesk Fusion 360 part; units mm, degrees
sketch "Boceto1" plane through (0, 0, 0) normal (0, 0, 1) x (1, 0, 0)
  circle A0 centre (0, 0) radius 2.5
  dimension "d1" = 5
  constraint coincident A0.centre origin
  measures "d1" diameter of A0
extrude "Extruir3" add sketch "Boceto1" along normal blind 150
